Autodesk Inventor part; units mm, degrees
(part 2 of 2)
hole "Hole3" at (3.5, -57.971, -9.3) at (4, -24.0349, -9.3) at (19.873, -45.2549, -9.3) at (19.85, -9.75, -9.3) at (9.85, -9.75, -9.3) at (17.9752, -23, -9.3) direction (0, 0, 1) diameter 4 depth 5.5 counterbore diameter 4.5 counterbore depth 0.5
sketch "Sketch6" plane through (0, -65.8371, 0) normal (-1, 0, 0) x (0, 0, 1)
  circle A0 centre (2, 25.6685) radius 1.75 projected
  circle A1 centre (2, 35.6685) radius 1.75 projected
  line L0 (0, 43.4488) -> (4, 43.4488) projected
  line L1 (0, 43.4488) -> (0, 17.8883) projected
  line L2 (0, 17.8883) -> (4, 17.8883) projected
  line L3 (4, 43.4488) -> (4, 17.8883) projected
  point P0 (0, 65.8371)
hole "Hole4" at (0, -40.1685, 2) at (0, -30.1685, 2) direction (1, 0, 0) diameter 2.9 end through all countersink diameter 6 countersink angle 90 clearance for "Countersunk Flat Head Screw ISO 2009/7046" size "M2.5" standard "ISO"
sketch "Sketch8" plane through (27.4, -6.5, -9.3) normal (1, 0, 0) x (0, 0, -1)
  line L0 (-6.3, 2.228) -> (-6.3, 0) projected
  line L1 (-6.3, 0) -> (0, 0) projected
  line L2 (0, 0) -> (0, 6.5) projected
  line L3 (-9.3, 6.5) -> (0, 6.5) projected
  line L4 (-9.3, 2.228) -> (-9.3, 6.5) projected
  line L5 (-9.3, 2.228) -> (-6.3, 2.228) projected
  line L6 (-6.3, 0) -> (0, 6.5)
  point P0 (-9.3, 6.5)
  point P1 (-3.15, 3.25)
  constraints: 2 end point, 1 midpoint
hole "Hole6" at (27.4, -3.25, -6.15) direction (-1, 0, 0) diameter 4 depth 6.5 counterbore diameter 4.5 counterbore depth 0.5
sketch "Sketch9" plane through (23.1, -65.8371, -9.3) normal (1, 0, 0) x (0, 0, -1)
  line L0 (-6.3, 57.1475) -> (-9.3, 57.1475) projected
  line L1 (-9.3, 48.6622) -> (-9.3, 57.1475) projected
  line L2 (-9.3, 48.6622) -> (-6.3, 48.6622) projected
  line L3 (-9.3, 57.1475) -> (0, 57.1475)
  line L4 (0, 57.1475) -> (0, 48.6622)
  line L5 (0, 48.6622) -> (-9.3, 48.6622)
  line L6 (-9.3, 48.6622) -> (-9.3, 57.1475)
  line L7 (-6.3, 41.8802) -> (-9.3, 41.8802) projected
  line L8 (-9.3, 0) -> (-9.3, 41.8802) projected
  line L9 (-9.3, 0) -> (0, 0) projected
  line L10 (0, 0) -> (0, 59.3371) projected
  line L11 (-6.3, 59.3371) -> (0, 59.3371) projected
  line L12 (-6.3, 59.3371) -> (-6.3, 57.1475) projected
  line L13 (-6.3, 57.1475) -> (-9.3, 57.1475) projected
  line L14 (-9.3, 48.6622) -> (-9.3, 57.1475) projected
  line L15 (-9.3, 48.6622) -> (-6.3, 48.6622) projected
  line L16 (-6.3, 48.6622) -> (-6.3, 41.8802) projected
  circle A0 centre (-4.3, 52.4871) radius 2.75
  circle A1 centre (-6.55, 2.75) radius 2.75
  circle A2 centre (-4.3, 52.4871) radius 2
  line L17 (-5.5, 54.0871) -> (-5.5, 58.0871) projected
  line L18 (-6.3, 46.1371) -> (-6.3, 56.1371) projected
  point P0 (-9.3, 65.8371)
  dimension "d174" = 4
  dimension "d165" = 5.5
  dimension "d173" = 5.5
  constraints: 8 end point, 2 centre point, 2 parallel, 2 point on line, 2 tangent, 1 coincident, 1 horizontal, 1 perpendicular, 1 vertical, 3 other
  measures "d165" diameter of A0
  measures "d173" diameter of A1
hole "Hole7" at (23.1, -13.35, -5) at (23.1, -63.0871, -2.75) direction (-1, 0, 0) diameter 3 depth 5 counterbore diameter 3.5 counterbore depth 0.5
sketch "Sketch10" plane through (9.002, -47.4193, -1.6) normal (0, 0, -1) x (-1, 0, 0)
  circle A0 centre (0, 0) radius 4.6 projected
  circle A1 centre (0, 0) radius 1.25
  point P0 (9.002, 47.4193)
  dimension "d175" = 2.5
  constraints: 1 centre point, 1 coincident
  measures "d175" diameter of A1
extrude "Extrusion11" cut sketch "Sketch10" against normal blind 1.4 contours A1
body "Solid1"
